Autodesk Inventor part; units mm, degrees
(part 12 of 13)
  spline S1673 degree 3 poles (16.8571, 16.1547) (16.6103, 16.1547) (16.4102, 15.9546) (16.4102, 15.7078) knots 0 0 0 0 1 1 1 1
  line L5245 (16.8571, 16.1547) -> (16.6103, 16.1547) construction
  line L5246 (16.6103, 16.1547) -> (16.4102, 15.9546) construction
  line L5247 (16.4102, 15.9546) -> (16.4102, 15.7078) construction
  spline S1674 degree 3 poles (16.4102, 15.7078) (16.4102, 15.461) (16.6103, 15.2608) (16.8571, 15.2608) knots 0 0 0 0 1 1 1 1
  line L5248 (16.4102, 15.7078) -> (16.4102, 15.461) construction
  line L5249 (16.4102, 15.461) -> (16.6103, 15.2608) construction
  line L5250 (16.6103, 15.2608) -> (16.8571, 15.2608) construction
  spline S1675 degree 3 poles (16.8571, 15.2608) (17.1039, 15.2608) (17.3041, 15.461) (17.3041, 15.7078) knots 0 0 0 0 1 1 1 1
  line L5251 (16.8571, 15.2608) -> (17.1039, 15.2608) construction
  line L5252 (17.1039, 15.2608) -> (17.3041, 15.461) construction
  line L5253 (17.3041, 15.461) -> (17.3041, 15.7078) construction
  spline S1676 degree 3 poles (17.3041, 18.2619) (17.3041, 18.5087) (17.1039, 18.7088) (16.8571, 18.7088) knots 0 0 0 0 1 1 1 1
  line L5254 (17.3041, 18.2619) -> (17.3041, 18.5087) construction
  line L5255 (17.3041, 18.5087) -> (17.1039, 18.7088) construction
  line L5256 (17.1039, 18.7088) -> (16.8571, 18.7088) construction
  spline S1677 degree 3 poles (16.8571, 18.7088) (16.6103, 18.7088) (16.4102, 18.5087) (16.4102, 18.2619) knots 0 0 0 0 1 1 1 1
  line L5257 (16.8571, 18.7088) -> (16.6103, 18.7088) construction
  line L5258 (16.6103, 18.7088) -> (16.4102, 18.5087) construction
  line L5259 (16.4102, 18.5087) -> (16.4102, 18.2619) construction
  spline S1678 degree 3 poles (16.4102, 18.2619) (16.4102, 18.0151) (16.6103, 17.8149) (16.8571, 17.8149) knots 0 0 0 0 1 1 1 1
  line L5260 (16.4102, 18.2619) -> (16.4102, 18.0151) construction
  line L5261 (16.4102, 18.0151) -> (16.6103, 17.8149) construction
  line L5262 (16.6103, 17.8149) -> (16.8571, 17.8149) construction
  spline S1679 degree 3 poles (16.8571, 17.8149) (17.1039, 17.8149) (17.3041, 18.0151) (17.3041, 18.2619) knots 0 0 0 0 1 1 1 1
  line L5263 (16.8571, 17.8149) -> (17.1039, 17.8149) construction
  line L5264 (17.1039, 17.8149) -> (17.3041, 18.0151) construction
  line L5265 (17.3041, 18.0151) -> (17.3041, 18.2619) construction
  spline S1680 degree 3 poles (17.3041, 20.816) (17.3041, 21.0628) (17.1039, 21.2629) (16.8571, 21.2629) knots 0 0 0 0 1 1 1 1
  line L5266 (17.3041, 20.816) -> (17.3041, 21.0628) construction
  line L5267 (17.3041, 21.0628) -> (17.1039, 21.2629) construction
  line L5268 (17.1039, 21.2629) -> (16.8571, 21.2629) construction
  spline S1681 degree 3 poles (16.8571, 21.2629) (16.6103, 21.2629) (16.4102, 21.0628) (16.4102, 20.816) knots 0 0 0 0 1 1 1 1
  line L5269 (16.8571, 21.2629) -> (16.6103, 21.2629) construction
  line L5270 (16.6103, 21.2629) -> (16.4102, 21.0628) construction
  line L5271 (16.4102, 21.0628) -> (16.4102, 20.816) construction
  spline S1682 degree 3 poles (16.4102, 20.816) (16.4102, 20.5692) (16.6103, 20.369) (16.8571, 20.369) knots 0 0 0 0 1 1 1 1
  line L5272 (16.4102, 20.816) -> (16.4102, 20.5692) construction
  line L5273 (16.4102, 20.5692) -> (16.6103, 20.369) construction
  line L5274 (16.6103, 20.369) -> (16.8571, 20.369) construction
  spline S1683 degree 3 poles (16.8571, 20.369) (17.1039, 20.369) (17.3041, 20.5692) (17.3041, 20.816) knots 0 0 0 0 1 1 1 1
  line L5275 (16.8571, 20.369) -> (17.1039, 20.369) construction
  line L5276 (17.1039, 20.369) -> (17.3041, 20.5692) construction
  line L5277 (17.3041, 20.5692) -> (17.3041, 20.816) construction
  spline S1684 degree 3 poles (19.8582, 13.1537) (19.8582, 13.4005) (19.658, 13.6006) (19.4112, 13.6006) knots 0 0 0 0 1 1 1 1
  line L5278 (19.8582, 13.1537) -> (19.8582, 13.4005) construction
  line L5279 (19.8582, 13.4005) -> (19.658, 13.6006) construction
  line L5280 (19.658, 13.6006) -> (19.4112, 13.6006) construction
  spline S1685 degree 3 poles (19.4112, 13.6006) (19.1644, 13.6006) (18.9643, 13.4005) (18.9643, 13.1537) knots 0 0 0 0 1 1 1 1
  line L5281 (19.4112, 13.6006) -> (19.1644, 13.6006) construction
  line L5282 (19.1644, 13.6006) -> (18.9643, 13.4005) construction
  line L5283 (18.9643, 13.4005) -> (18.9643, 13.1537) construction
  spline S1686 degree 3 poles (18.9643, 13.1537) (18.9643, 12.9069) (19.1644, 12.7067) (19.4112, 12.7067) knots 0 0 0 0 1 1 1 1
  line L5284 (18.9643, 13.1537) -> (18.9643, 12.9069) construction
  line L5285 (18.9643, 12.9069) -> (19.1644, 12.7067) construction
  line L5286 (19.1644, 12.7067) -> (19.4112, 12.7067) construction
  spline S1687 degree 3 poles (19.4112, 12.7067) (19.658, 12.7067) (19.8582, 12.9069) (19.8582, 13.1537) knots 0 0 0 0 1 1 1 1
  line L5287 (19.4112, 12.7067) -> (19.658, 12.7067) construction
  line L5288 (19.658, 12.7067) -> (19.8582, 12.9069) construction
  line L5289 (19.8582, 12.9069) -> (19.8582, 13.1537) construction
  spline S1688 degree 3 poles (19.8582, 15.7078) (19.8582, 15.9546) (19.658, 16.1547) (19.4112, 16.1547) knots 0 0 0 0 1 1 1 1
  line L5290 (19.8582, 15.7078) -> (19.8582, 15.9546) construction
  line L5291 (19.8582, 15.9546) -> (19.658, 16.1547) construction
  line L5292 (19.658, 16.1547) -> (19.4112, 16.1547) construction
  spline S1689 degree 3 poles (19.4112, 16.1547) (19.1644, 16.1547) (18.9643, 15.9546) (18.9643, 15.7078) knots 0 0 0 0 1 1 1 1
  line L5293 (19.4112, 16.1547) -> (19.1644, 16.1547) construction
  line L5294 (19.1644, 16.1547) -> (18.9643, 15.9546) construction
  line L5295 (18.9643, 15.9546) -> (18.9643, 15.7078) construction
  spline S1690 degree 3 poles (18.9643, 15.7078) (18.9643, 15.461) (19.1644, 15.2608) (19.4112, 15.2608) knots 0 0 0 0 1 1 1 1
  line L5296 (18.9643, 15.7078) -> (18.9643, 15.461) construction
  line L5297 (18.9643, 15.461) -> (19.1644, 15.2608) construction
  line L5298 (19.1644, 15.2608) -> (19.4112, 15.2608) construction
  spline S1691 degree 3 poles (19.4112, 15.2608) (19.658, 15.2608) (19.8582, 15.461) (19.8582, 15.7078) knots 0 0 0 0 1 1 1 1
  line L5299 (19.4112, 15.2608) -> (19.658, 15.2608) construction
  line L5300 (19.658, 15.2608) -> (19.8582, 15.461) construction
  line L5301 (19.8582, 15.461) -> (19.8582, 15.7078) construction
  spline S1692 degree 3 poles (19.8582, 18.2619) (19.8582, 18.5087) (19.658, 18.7088) (19.4112, 18.7088) knots 0 0 0 0 1 1 1 1
  line L5302 (19.8582, 18.2619) -> (19.8582, 18.5087) construction
  line L5303 (19.8582, 18.5087) -> (19.658, 18.7088) construction
  line L5304 (19.658, 18.7088) -> (19.4112, 18.7088) construction
  spline S1693 degree 3 poles (19.4112, 18.7088) (19.1644, 18.7088) (18.9643, 18.5087) (18.9643, 18.2619) knots 0 0 0 0 1 1 1 1
  line L5305 (19.4112, 18.7088) -> (19.1644, 18.7088) construction
  line L5306 (19.1644, 18.7088) -> (18.9643, 18.5087) construction
  line L5307 (18.9643, 18.5087) -> (18.9643, 18.2619) construction
  spline S1694 degree 3 poles (18.9643, 18.2619) (18.9643, 18.0151) (19.1644, 17.8149) (19.4112, 17.8149) knots 0 0 0 0 1 1 1 1
  line L5308 (18.9643, 18.2619) -> (18.9643, 18.0151) construction
  line L5309 (18.9643, 18.0151) -> (19.1644, 17.8149) construction
  line L5310 (19.1644, 17.8149) -> (19.4112, 17.8149) construction
  spline S1695 degree 3 poles (19.4112, 17.8149) (19.658, 17.8149) (19.8582, 18.0151) (19.8582, 18.2619) knots 0 0 0 0 1 1 1 1
  line L5311 (19.4112, 17.8149) -> (19.658, 17.8149) construction
  line L5312 (19.658, 17.8149) -> (19.8582, 18.0151) construction
  line L5313 (19.8582, 18.0151) -> (19.8582, 18.2619) construction
  spline S1696 degree 3 poles (19.8582, 20.816) (19.8582, 21.0628) (19.658, 21.2629) (19.4112, 21.2629) knots 0 0 0 0 1 1 1 1
  line L5314 (19.8582, 20.816) -> (19.8582, 21.0628) construction
  line L5315 (19.8582, 21.0628) -> (19.658, 21.2629) construction
  line L5316 (19.658, 21.2629) -> (19.4112, 21.2629) construction
  spline S1697 degree 3 poles (19.4112, 21.2629) (19.1644, 21.2629) (18.9643, 21.0628) (18.9643, 20.816) knots 0 0 0 0 1 1 1 1
  line L5317 (19.4112, 21.2629) -> (19.1644, 21.2629) construction
  line L5318 (19.1644, 21.2629) -> (18.9643, 21.0628) construction
  line L5319 (18.9643, 21.0628) -> (18.9643, 20.816) construction
  spline S1698 degree 3 poles (18.9643, 20.816) (18.9643, 20.5692) (19.1644, 20.369) (19.4112, 20.369) knots 0 0 0 0 1 1 1 1
  line L5320 (18.9643, 20.816) -> (18.9643, 20.5692) construction
  line L5321 (18.9643, 20.5692) -> (19.1644, 20.369) construction
  line L5322 (19.1644, 20.369) -> (19.4112, 20.369) construction
  spline S1699 degree 3 poles (19.4112, 20.369) (19.658, 20.369) (19.8582, 20.5692) (19.8582, 20.816) knots 0 0 0 0 1 1 1 1
  line L5323 (19.4112, 20.369) -> (19.658, 20.369) construction
  line L5324 (19.658, 20.369) -> (19.8582, 20.5692) construction
  line L5325 (19.8582, 20.5692) -> (19.8582, 20.816) construction
  spline S1700 degree 3 poles (4.0865, 32.1817) (4.0865, 32.8164) (3.5719, 33.3312) (2.9373, 33.3312) knots 0 0 0 0 1 1 1 1
  line L5326 (4.0865, 32.1817) -> (4.0865, 32.8164) construction
  line L5327 (4.0865, 32.8164) -> (3.5719, 33.3312) construction
  line L5328 (3.5719, 33.3312) -> (2.9373, 33.3312) construction
  spline S1701 degree 3 poles (2.9373, 33.3312) (2.3026, 33.3312) (1.7878, 32.8164) (1.7878, 32.1817) knots 0 0 0 0 1 1 1 1
  line L5329 (2.9373, 33.3312) -> (2.3026, 33.3312) construction
  line L5330 (2.3026, 33.3312) -> (1.7878, 32.8164) construction
  line L5331 (1.7878, 32.8164) -> (1.7878, 32.1817) construction
  spline S1702 degree 3 poles (1.7878, 32.1817) (1.7878, 31.5471) (2.3026, 31.0325) (2.9373, 31.0325) knots 0 0 0 0 1 1 1 1
  line L5332 (1.7878, 32.1817) -> (1.7878, 31.5471) construction
  line L5333 (1.7878, 31.5471) -> (2.3026, 31.0325) construction
  line L5334 (2.3026, 31.0325) -> (2.9373, 31.0325) construction
  spline S1703 degree 3 poles (2.9373, 31.0325) (3.5719, 31.0325) (4.0865, 31.5471) (4.0865, 32.1817) knots 0 0 0 0 1 1 1 1
  line L5335 (2.9373, 31.0325) -> (3.5719, 31.0325) construction
  line L5336 (3.5719, 31.0325) -> (4.0865, 31.5471) construction
  line L5337 (4.0865, 31.5471) -> (4.0865, 32.1817) construction
  spline S1704 degree 3 poles (4.0865, 1.7878) (4.0865, 2.4225) (3.5719, 2.9373) (2.9373, 2.9373) knots 0 0 0 0 1 1 1 1
  line L5338 (4.0865, 1.7878) -> (4.0865, 2.4225) construction
  line L5339 (4.0865, 2.4225) -> (3.5719, 2.9373) construction
  line L5340 (3.5719, 2.9373) -> (2.9373, 2.9373) construction
  spline S1705 degree 3 poles (2.9373, 2.9373) (2.3026, 2.9373) (1.7878, 2.4225) (1.7878, 1.7878) knots 0 0 0 0 1 1 1 1
  line L5341 (2.9373, 2.9373) -> (2.3026, 2.9373) construction
  line L5342 (2.3026, 2.9373) -> (1.7878, 2.4225) construction
  line L5343 (1.7878, 2.4225) -> (1.7878, 1.7878) construction
  spline S1706 degree 3 poles (1.7878, 1.7878) (1.7878, 1.1532) (2.3026, 0.6385) (2.9373, 0.6385) knots 0 0 0 0 1 1 1 1
  line L5344 (1.7878, 1.7878) -> (1.7878, 1.1532) construction
  line L5345 (1.7878, 1.1532) -> (2.3026, 0.6385) construction
  line L5346 (2.3026, 0.6385) -> (2.9373, 0.6385) construction
  spline S1707 degree 3 poles (2.9373, 0.6385) (3.5719, 0.6385) (4.0865, 1.1532) (4.0865, 1.7878) knots 0 0 0 0 1 1 1 1
  line L5347 (2.9373, 0.6385) -> (3.5719, 0.6385) construction
  line L5348 (3.5719, 0.6385) -> (4.0865, 1.1532) construction
  line L5349 (4.0865, 1.1532) -> (4.0865, 1.7878) construction
  spline S1708 degree 3 poles (52.3592, 1.7878) (52.3592, 2.4225) (51.8445, 2.9373) (51.2099, 2.9373) knots 0 0 0 0 1 1 1 1
  line L5350 (52.3592, 1.7878) -> (52.3592, 2.4225) construction
  line L5351 (52.3592, 2.4225) -> (51.8445, 2.9373) construction
  line L5352 (51.8445, 2.9373) -> (51.2099, 2.9373) construction
  spline S1709 degree 3 poles (51.2099, 2.9373) (50.5753, 2.9373) (50.0605, 2.4225) (50.0605, 1.7878) knots 0 0 0 0 1 1 1 1
  line L5353 (51.2099, 2.9373) -> (50.5753, 2.9373) construction
  line L5354 (50.5753, 2.9373) -> (50.0605, 2.4225) construction
  line L5355 (50.0605, 2.4225) -> (50.0605, 1.7878) construction
  spline S1710 degree 3 poles (50.0605, 1.7878) (50.0605, 1.1532) (50.5753, 0.6385) (51.2099, 0.6385) knots 0 0 0 0 1 1 1 1
  line L5356 (50.0605, 1.7878) -> (50.0605, 1.1532) construction
  line L5357 (50.0605, 1.1532) -> (50.5753, 0.6385) construction
  line L5358 (50.5753, 0.6385) -> (51.2099, 0.6385) construction
  spline S1711 degree 3 poles (51.2099, 0.6385) (51.8445, 0.6385) (52.3592, 1.1532) (52.3592, 1.7878) knots 0 0 0 0 1 1 1 1
  line L5359 (51.2099, 0.6385) -> (51.8445, 0.6385) construction
  line L5360 (51.8445, 0.6385) -> (52.3592, 1.1532) construction
  line L5361 (52.3592, 1.1532) -> (52.3592, 1.7878) construction
  spline S1712 degree 3 poles (52.3592, 32.1817) (52.3592, 32.8164) (51.8445, 33.3312) (51.2099, 33.3312) knots 0 0 0 0 1 1 1 1
  line L5362 (52.3592, 32.1817) -> (52.3592, 32.8164) construction
  line L5363 (52.3592, 32.8164) -> (51.8445, 33.3312) construction
  line L5364 (51.8445, 33.3312) -> (51.2099, 33.3312) construction
  spline S1713 degree 3 poles (51.2099, 33.3312) (50.5753, 33.3312) (50.0605, 32.8164) (50.0605, 32.1817) knots 0 0 0 0 1 1 1 1
  line L5365 (51.2099, 33.3312) -> (50.5753, 33.3312) construction
  line L5366 (50.5753, 33.3312) -> (50.0605, 32.8164) construction
  line L5367 (50.0605, 32.8164) -> (50.0605, 32.1817) construction
  spline S1714 degree 3 poles (50.0605, 32.1817) (50.0605, 31.5471) (50.5753, 31.0325) (51.2099, 31.0325) knots 0 0 0 0 1 1 1 1
  line L5368 (50.0605, 32.1817) -> (50.0605, 31.5471) construction
  line L5369 (50.0605, 31.5471) -> (50.5753, 31.0325) construction
  line L5370 (50.5753, 31.0325) -> (51.2099, 31.0325) construction
  spline S1715 degree 3 poles (51.2099, 31.0325) (51.8445, 31.0325) (52.3592, 31.5471) (52.3592, 32.1817) knots 0 0 0 0 1 1 1 1
  line L5371 (51.2099, 31.0325) -> (51.8445, 31.0325) construction
  line L5372 (51.8445, 31.0325) -> (52.3592, 31.5471) construction
  line L5373 (52.3592, 31.5471) -> (52.3592, 32.1817) construction
  line L5374 (23.6255, 14.4308) -> (23.6255, 14.1754)
  line L5375 (20.6882, 31.0325) -> (20.6882, 2.9373)
  line L5376 (18.1341, 31.0325) -> (18.1341, 2.9373)
  line L5377 (24.5194, 10.0887) -> (24.9026, 9.7057)
  line L5378 (25.6689, 10.3442) -> (26.3074, 9.7057)
  line L5379 (21.8377, 10.0887) -> (24.5194, 10.0887)
  line L5380 (21.9653, 10.3442) -> (25.6689, 10.3442)
  line L5381 (21.7099, 9.8333) -> (22.7316, 9.8333)
  line L5382 (20.6882, 10.855) -> (21.7099, 9.8333)
  line L5383 (20.4329, 10.855) -> (20.6882, 10.855)
  line L5384 (20.9436, 10.9827) -> (21.8377, 10.0887)
  line L5385 (20.9436, 12.8983) -> (20.9436, 10.9827)
  line L5386 (21.1992, 11.1103) -> (21.9653, 10.3442)
  line L5387 (20.6882, 13.1537) -> (20.9436, 12.8983)
  line L5388 (20.4329, 13.1537) -> (20.6882, 13.1537)
  line L5389 (21.1992, 15.4524) -> (21.1992, 11.1103)
  line L5390 (20.9436, 15.7078) -> (21.1992, 15.4524)
  line L5391 (20.4329, 15.7078) -> (20.9436, 15.7078)
  line L5392 (20.6882, 25.9242) -> (21.1992, 25.4133)
  line L5393 (20.4329, 25.9242) -> (20.6882, 25.9242)
  line L5394 (33.4588, 31.0325) -> (33.4588, 2.9373)
  line L5395 (36.0129, 31.0325) -> (36.0129, 2.9373)
  line L5396 (22.7316, 20.4329) -> (22.8592, 20.3051)
  line L5397 (24.6472, 20.6882) -> (24.9026, 20.4329)
  line L5398 (21.4546, 20.6882) -> (24.6472, 20.6882)
  line L5399 (21.3268, 20.4329) -> (22.7316, 20.4329)
  line L5400 (20.6882, 21.0714) -> (21.3268, 20.4329)
  line L5401 (20.4329, 21.0714) -> (20.6882, 21.0714)
  line L5402 (20.9436, 21.1992) -> (21.4546, 20.6882)
  line L5403 (25.9242, 20.9436) -> (26.3074, 20.5606)
  line L5404 (21.5822, 20.9436) -> (25.9242, 20.9436)
  line L5405 (20.9436, 23.1148) -> (20.9436, 21.1992)
  line L5406 (21.1992, 21.3268) -> (21.5822, 20.9436)
  line L5407 (21.1992, 25.4133) -> (21.1992, 21.3268)
  line L5408 (20.6882, 23.3701) -> (20.9436, 23.1148)
  spline S1716 degree 3 poles (19.4112, 32.3095) (20.1164, 32.3095) (20.6882, 31.7376) (20.6882, 31.0325) knots 0 0 0 0 1 1 1 1
  line L5409 (19.4112, 32.3095) -> (20.1164, 32.3095) construction
  line L5410 (20.1164, 32.3095) -> (20.6882, 31.7376) construction
  line L5411 (20.6882, 31.7376) -> (20.6882, 31.0325) construction
  spline S1717 degree 3 poles (18.1341, 31.0325) (18.1341, 31.7376) (18.706, 32.3095) (19.4112, 32.3095) knots 0 0 0 0 1 1 1 1
  line L5412 (18.1341, 31.0325) -> (18.1341, 31.7376) construction
  line L5413 (18.1341, 31.7376) -> (18.706, 32.3095) construction
  line L5414 (18.706, 32.3095) -> (19.4112, 32.3095) construction
  spline S1718 degree 3 poles (19.4112, 32.0541) (19.9753, 32.0541) (20.4329, 31.5966) (20.4329, 31.0325) knots 0 0 0 0 1 1 1 1
  line L5415 (19.4112, 32.0541) -> (19.9753, 32.0541) construction
  line L5416 (19.9753, 32.0541) -> (20.4329, 31.5966) construction
  line L5417 (20.4329, 31.5966) -> (20.4329, 31.0325) construction
  spline S1719 degree 3 poles (19.4112, 29.5) (19.9753, 29.5) (20.4329, 29.0425) (20.4329, 28.4784) knots 0 0 0 0 1 1 1 1
  line L5418 (19.4112, 29.5) -> (19.9753, 29.5) construction
  line L5419 (19.9753, 29.5) -> (20.4329, 29.0425) construction
  line L5420 (20.4329, 29.0425) -> (20.4329, 28.4784) construction
  spline S1720 degree 3 poles (20.4329, 28.4784) (20.4329, 27.9142) (19.9753, 27.4567) (19.4112, 27.4567) knots 0 0 0 0 1 1 1 1
  line L5421 (20.4329, 28.4784) -> (20.4329, 27.9142) construction
  line L5422 (20.4329, 27.9142) -> (19.9753, 27.4567) construction
  line L5423 (19.9753, 27.4567) -> (19.4112, 27.4567) construction
  spline S1721 degree 3 poles (20.4329, 31.0325) (20.4329, 30.4683) (19.9753, 30.0108) (19.4112, 30.0108) knots 0 0 0 0 1 1 1 1
  line L5424 (20.4329, 31.0325) -> (20.4329, 30.4683) construction
  line L5425 (20.4329, 30.4683) -> (19.9753, 30.0108) construction
  line L5426 (19.9753, 30.0108) -> (19.4112, 30.0108) construction
  spline S1722 degree 3 poles (33.4588, 31.0325) (33.4588, 31.7376) (34.0307, 32.3095) (34.7358, 32.3095) knots 0 0 0 0 1 1 1 1
  line L5427 (33.4588, 31.0325) -> (33.4588, 31.7376) construction
  line L5428 (33.4588, 31.7376) -> (34.0307, 32.3095) construction
  line L5429 (34.0307, 32.3095) -> (34.7358, 32.3095) construction
  spline S1723 degree 3 poles (34.7358, 32.3095) (35.441, 32.3095) (36.0129, 31.7376) (36.0129, 31.0325) knots 0 0 0 0 1 1 1 1
  line L5430 (34.7358, 32.3095) -> (35.441, 32.3095) construction
  line L5431 (35.441, 32.3095) -> (36.0129, 31.7376) construction
  line L5432 (36.0129, 31.7376) -> (36.0129, 31.0325) construction
  spline S1724 degree 3 poles (34.7358, 30.0108) (34.1717, 30.0108) (33.7142, 30.4683) (33.7142, 31.0325) knots 0 0 0 0 1 1 1 1
  line L5433 (34.7358, 30.0108) -> (34.1717, 30.0108) construction
  line L5434 (34.1717, 30.0108) -> (33.7142, 30.4683) construction
  line L5435 (33.7142, 30.4683) -> (33.7142, 31.0325) construction
  spline S1725 degree 3 poles (33.7142, 31.0325) (33.7142, 31.5966) (34.1717, 32.0541) (34.7358, 32.0541) knots 0 0 0 0 1 1 1 1
  line L5436 (33.7142, 31.0325) -> (33.7142, 31.5966) construction
  line L5437 (33.7142, 31.5966) -> (34.1717, 32.0541) construction
  line L5438 (34.1717, 32.0541) -> (34.7358, 32.0541) construction
  spline S1726 degree 3 poles (34.7358, 22.3485) (34.1717, 22.3485) (33.7142, 22.806) (33.7142, 23.3701) knots 0 0 0 0 1 1 1 1
  line L5439 (34.7358, 22.3485) -> (34.1717, 22.3485) construction
  line L5440 (34.1717, 22.3485) -> (33.7142, 22.806) construction
  line L5441 (33.7142, 22.806) -> (33.7142, 23.3701) construction
  spline S1727 degree 3 poles (33.7142, 23.3701) (33.7142, 23.9342) (34.1717, 24.3918) (34.7358, 24.3918) knots 0 0 0 0 1 1 1 1
  line L5442 (33.7142, 23.3701) -> (33.7142, 23.9342) construction
  line L5443 (33.7142, 23.9342) -> (34.1717, 24.3918) construction
  line L5444 (34.1717, 24.3918) -> (34.7358, 24.3918) construction
  spline S1728 degree 3 poles (34.7358, 19.7943) (34.1717, 19.7943) (33.7142, 20.2519) (33.7142, 20.816) knots 0 0 0 0 1 1 1 1
  line L5445 (34.7358, 19.7943) -> (34.1717, 19.7943) construction
  line L5446 (34.1717, 19.7943) -> (33.7142, 20.2519) construction
  line L5447 (33.7142, 20.2519) -> (33.7142, 20.816) construction
  spline S1729 degree 3 poles (33.7142, 20.816) (33.7142, 21.3801) (34.1717, 21.8377) (34.7358, 21.8377) knots 0 0 0 0 1 1 1 1
  line L5448 (33.7142, 20.816) -> (33.7142, 21.3801) construction
  line L5449 (33.7142, 21.3801) -> (34.1717, 21.8377) construction
  line L5450 (34.1717, 21.8377) -> (34.7358, 21.8377) construction
  spline S1730 degree 3 poles (34.7358, 14.6861) (34.1717, 14.6861) (33.7142, 15.1437) (33.7142, 15.7078) knots 0 0 0 0 1 1 1 1
  line L5451 (34.7358, 14.6861) -> (34.1717, 14.6861) construction
  line L5452 (34.1717, 14.6861) -> (33.7142, 15.1437) construction
  line L5453 (33.7142, 15.1437) -> (33.7142, 15.7078) construction
  spline S1731 degree 3 poles (33.7142, 15.7078) (33.7142, 16.2719) (34.1717, 16.7295) (34.7358, 16.7295) knots 0 0 0 0 1 1 1 1
  line L5454 (33.7142, 15.7078) -> (33.7142, 16.2719) construction
  line L5455 (33.7142, 16.2719) -> (34.1717, 16.7295) construction
  line L5456 (34.1717, 16.7295) -> (34.7358, 16.7295) construction
  spline S1732 degree 3 poles (20.6882, 2.9373) (20.6882, 2.2321) (20.1164, 1.6602) (19.4112, 1.6602) knots 0 0 0 0 1 1 1 1
  line L5457 (20.6882, 2.9373) -> (20.6882, 2.2321) construction
  line L5458 (20.6882, 2.2321) -> (20.1164, 1.6602) construction
  line L5459 (20.1164, 1.6602) -> (19.4112, 1.6602) construction
  spline S1733 degree 3 poles (19.4112, 1.6602) (18.706, 1.6602) (18.1341, 2.2321) (18.1341, 2.9373) knots 0 0 0 0 1 1 1 1
  line L5460 (19.4112, 1.6602) -> (18.706, 1.6602) construction
  line L5461 (18.706, 1.6602) -> (18.1341, 2.2321) construction
  line L5462 (18.1341, 2.2321) -> (18.1341, 2.9373) construction
  spline S1734 degree 3 poles (34.7358, 1.6602) (34.0307, 1.6602) (33.4588, 2.2321) (33.4588, 2.9373) knots 0 0 0 0 1 1 1 1
  line L5463 (34.7358, 1.6602) -> (34.0307, 1.6602) construction
  line L5464 (34.0307, 1.6602) -> (33.4588, 2.2321) construction
  line L5465 (33.4588, 2.2321) -> (33.4588, 2.9373) construction
  spline S1735 degree 3 poles (36.0129, 2.9373) (36.0129, 2.2321) (35.441, 1.6602) (34.7358, 1.6602) knots 0 0 0 0 1 1 1 1
  line L5466 (36.0129, 2.9373) -> (36.0129, 2.2321) construction
  line L5467 (36.0129, 2.2321) -> (35.441, 1.6602) construction
  line L5468 (35.441, 1.6602) -> (34.7358, 1.6602) construction
  line L5469 (20.4329, 23.3701) -> (20.6882, 23.3701)
  line L5470 (27.1247, 13.7922) -> (26.5116, 13.7922)
  line L5471 (27.3289, 13.9352) -> (27.1247, 13.7922)
  line L5472 (27.3289, 14.16) -> (27.3289, 13.9352)
  line L5473 (27.1247, 14.303) -> (27.3289, 14.16)
  line L5474 (27.1247, 14.303) -> (26.5116, 14.303)
  line L5475 (26.9203, 14.303) -> (26.9203, 13.7922)
  line L5476 (27.3289, 14.9569) -> (26.8181, 14.5482)
  line L5477 (26.8181, 15.059) -> (26.8181, 14.5482)
  line L5478 (27.3289, 14.9569) -> (26.5116, 14.9569)
  line L5479 (27.1247, 21.7099) -> (26.5116, 21.7099)
  line L5480 (27.3289, 21.8529) -> (27.1247, 21.7099)
  line L5481 (27.3289, 22.0777) -> (27.3289, 21.8529)
  line L5482 (27.1247, 22.2207) -> (27.3289, 22.0777)
  line L5483 (27.1247, 22.2207) -> (26.5116, 22.2207)
  line L5484 (26.9203, 22.2207) -> (26.9203, 21.7099)
  line L5485 (27.3289, 22.9767) -> (26.5116, 22.5681)
  line L5486 (27.3289, 22.9767) -> (27.3289, 22.4659)
  line L5487 (27.1247, 24.264) -> (26.5116, 24.264)
  line L5488 (27.3289, 24.407) -> (27.1247, 24.264)
  line L5489 (27.3289, 24.6318) -> (27.3289, 24.407)
  line L5490 (27.1247, 24.7748) -> (27.3289, 24.6318)
  line L5491 (27.1247, 24.7748) -> (26.5116, 24.7748)
  line L5492 (26.9203, 24.7748) -> (26.9203, 24.264)
  line L5493 (27.2268, 25.4287) -> (27.3289, 25.3266)
  line L5494 (27.3289, 25.3266) -> (27.3289, 25.1222)
  line L5495 (27.3289, 25.1222) -> (27.2268, 25.0201)
  line L5496 (27.2268, 25.0201) -> (26.6137, 25.0201)
  line L5497 (26.5116, 25.1222) -> (26.6137, 25.0201)
  line L5498 (26.859, 25.4287) -> (26.9611, 25.3266)
  line L5499 (26.9611, 25.3266) -> (26.9611, 25.0201)
  line L5500 (26.5116, 25.3266) -> (26.5116, 25.1222)
  line L5501 (26.6137, 25.4287) -> (26.5116, 25.3266)
  line L5502 (26.859, 25.4287) -> (26.6137, 25.4287)
  line L5503 (21.8887, 17.751) -> (21.2758, 17.751)
  line L5504 (22.0931, 17.8942) -> (21.8887, 17.751)
  line L5505 (22.0931, 18.1189) -> (22.0931, 17.8942)
  line L5506 (21.8887, 18.2619) -> (22.0931, 18.1189)
  line L5507 (21.8887, 18.2619) -> (21.2758, 18.2619)
  line L5508 (21.6844, 18.2619) -> (21.6844, 17.751)
  line L5509 (22.0931, 18.6705) -> (21.9295, 18.507)
  line L5510 (22.0931, 18.6705) -> (21.2758, 18.6705)
  line L5511 (21.2758, 18.8136) -> (21.2758, 18.507)
  line L5512 (23.6766, 19.1558) -> (23.0636, 19.1558)
  line L5513 (23.8809, 19.2988) -> (23.6766, 19.1558)
  line L5514 (23.8809, 19.5236) -> (23.8809, 19.2988)
  line L5515 (23.6766, 19.6666) -> (23.8809, 19.5236)
  line L5516 (23.6766, 19.6666) -> (23.0636, 19.6666)
  line L5517 (23.4723, 19.6666) -> (23.4723, 19.1558)
  line L5518 (23.0636, 20.014) -> (23.1657, 19.9118)
  line L5519 (23.7788, 19.9118) -> (23.1657, 19.9118)
  line L5520 (23.8809, 20.014) -> (23.7788, 19.9118)
  line L5521 (23.8809, 20.2184) -> (23.8809, 20.014)
  line L5522 (23.7788, 20.3205) -> (23.8809, 20.2184)
  line L5523 (23.7788, 20.3205) -> (23.1657, 20.3205)
  line L5524 (23.1657, 20.3205) -> (23.0636, 20.2184)
  line L5525 (23.0636, 20.2184) -> (23.0636, 20.014)
  line L5526 (23.6766, 20.3205) -> (23.268, 19.9118)
  line L5527 (25.2857, 19.3193) -> (25.1222, 19.1558)
  line L5528 (25.2857, 19.3193) -> (24.4684, 19.3193)
  line L5529 (24.4684, 19.4623) -> (24.4684, 19.1558)
  line L5530 (25.2857, 19.8097) -> (25.1836, 19.7075)
  line L5531 (25.2857, 20.014) -> (25.2857, 19.8097)
  line L5532 (25.1836, 20.1161) -> (25.2857, 20.014)
  line L5533 (24.5706, 20.1161) -> (24.4684, 20.014)
  line L5534 (24.4684, 20.014) -> (24.4684, 19.8097)
  line L5535 (24.4684, 19.8097) -> (24.5706, 19.7075)
  line L5536 (24.918, 20.014) -> (24.918, 19.8097)
  line L5537 (25.1836, 20.1161) -> (25.0201, 20.1161)
  line L5538 (24.8157, 20.1161) -> (24.5706, 20.1161)
  line L5539 (24.918, 20.014) -> (24.8157, 20.1161)
  line L5540 (24.918, 20.014) -> (25.0201, 20.1161)
  line L5541 (26.6904, 19.3193) -> (26.527, 19.1558)
  line L5542 (26.6904, 19.3193) -> (25.8731, 19.3193)
  line L5543 (25.8731, 19.4623) -> (25.8731, 19.1558)
  line L5544 (26.6904, 19.8097) -> (26.5883, 19.7075)
  line L5545 (26.6904, 20.1161) -> (26.6904, 19.8097)
  line L5546 (26.5883, 20.2184) -> (26.6904, 20.1161)
  line L5547 (26.5883, 20.2184) -> (26.384, 20.2184)
  line L5548 (26.384, 20.2184) -> (25.8731, 19.7075)
  line L5549 (25.8731, 20.2184) -> (25.8731, 19.7075)
  line L5550 (22.0931, 30.8128) -> (21.9295, 30.6493)
  line L5551 (22.0931, 30.8128) -> (21.2758, 30.8128)
  line L5552 (21.2758, 30.9558) -> (21.2758, 30.6493)
  line L5553 (21.2758, 31.3032) -> (21.3779, 31.201)
  line L5554 (21.991, 31.201) -> (21.3779, 31.201)
  line L5555 (22.0931, 31.3032) -> (21.991, 31.201)
  line L5556 (22.0931, 31.5075) -> (22.0931, 31.3032)
  line L5557 (21.991, 31.6096) -> (22.0931, 31.5075)
  line L5558 (21.991, 31.6096) -> (21.3779, 31.6096)
  line L5559 (21.3779, 31.6096) -> (21.2758, 31.5075)
  line L5560 (21.2758, 31.5075) -> (21.2758, 31.3032)
  line L5561 (21.8887, 31.6096) -> (21.4801, 31.201)
  line L5562 (22.0931, 28.2587) -> (21.9295, 28.0952)
  line L5563 (22.0931, 28.2587) -> (21.2758, 28.2587)
  line L5564 (21.2758, 28.4017) -> (21.2758, 28.0952)
  line L5565 (22.0931, 28.8104) -> (21.9295, 28.6469)
  line L5566 (22.0931, 28.8104) -> (21.2758, 28.8104)
  line L5567 (21.2758, 28.9533) -> (21.2758, 28.6469)
  line L5568 (32.0541, 15.8611) -> (32.1562, 15.9632)
  line L5569 (32.0541, 15.8611) -> (32.0541, 15.6567)
  line L5570 (32.1562, 15.5545) -> (32.0541, 15.6567)
  line L5571 (32.7693, 15.5545) -> (32.8714, 15.6567)
  line L5572 (32.8714, 15.8611) -> (32.8714, 15.6567)
  line L5573 (32.8714, 15.8611) -> (32.7693, 15.9632)
  line L5574 (32.4219, 15.8611) -> (32.4219, 15.6567)
  line L5575 (32.3198, 15.5545) -> (32.1562, 15.5545)
  line L5576 (32.7693, 15.5545) -> (32.524, 15.5545)
  line L5577 (32.4219, 15.6567) -> (32.524, 15.5545)
  line L5578 (32.4219, 15.6567) -> (32.3198, 15.5545)
  line L5579 (32.0541, 18.1086) -> (32.5649, 18.5173)
  line L5580 (32.5649, 18.5173) -> (32.5649, 18.0065)
  line L5581 (32.8714, 18.1086) -> (32.0541, 18.1086)
  line L5582 (32.1562, 23.2169) -> (32.0541, 23.319)
  line L5583 (32.0541, 23.5234) -> (32.0541, 23.319)
  line L5584 (32.0541, 23.5234) -> (32.1562, 23.6255)
  line L5585 (32.7693, 23.6255) -> (32.1562, 23.6255)
  line L5586 (32.8714, 23.5234) -> (32.7693, 23.6255)
  line L5587 (32.524, 23.2169) -> (32.4219, 23.319)
  line L5588 (32.4219, 23.6255) -> (32.4219, 23.319)
  line L5589 (32.8714, 23.5234) -> (32.8714, 23.319)
  line L5590 (32.7693, 23.2169) -> (32.8714, 23.319)
  line L5591 (32.7693, 23.2169) -> (32.524, 23.2169)
  line L5592 (32.0541, 13.3069) -> (32.1562, 13.4091)
  line L5593 (32.0541, 13.3069) -> (32.0541, 13.0004)
  line L5594 (32.1562, 12.8983) -> (32.0541, 13.0004)
  line L5595 (32.3605, 12.8983) -> (32.1562, 12.8983)
  line L5596 (32.3605, 12.8983) -> (32.8714, 13.4091)
  line L5597 (32.8714, 13.4091) -> (32.8714, 12.8983)
  line L5598 (32.0541, 21.0714) -> (32.0541, 20.6627)
  line L5599 (32.4628, 21.0714) -> (32.0541, 21.0714)
  line L5600 (32.3605, 20.9693) -> (32.4628, 21.0714)
  line L5601 (32.3605, 20.9693) -> (32.3605, 20.7649)
  line L5602 (32.4628, 20.6627) -> (32.3605, 20.7649)
  line L5603 (32.7693, 20.6627) -> (32.4628, 20.6627)
  line L5604 (32.7693, 20.6627) -> (32.8714, 20.7649)
  line L5605 (32.8714, 20.9693) -> (32.8714, 20.7649)
  line L5606 (32.8714, 20.9693) -> (32.7693, 21.0714)
  line L5607 (32.0541, 25.6689) -> (32.8714, 26.0775)
  line L5608 (32.0541, 26.1796) -> (32.0541, 25.6689)
  line L5609 (32.8714, 28.6316) -> (32.7693, 28.7337)
  line L5610 (32.7693, 28.7337) -> (32.6058, 28.7337)
  line L5611 (32.4628, 28.5907) -> (32.6058, 28.7337)
  line L5612 (32.4628, 28.5907) -> (32.4628, 28.4681)
  line L5613 (32.6058, 28.3251) -> (32.4628, 28.4681)
  line L5614 (32.7693, 28.3251) -> (32.6058, 28.3251)
  line L5615 (32.7693, 28.3251) -> (32.8714, 28.4272)
  line L5616 (32.8714, 28.6316) -> (32.8714, 28.4272)
  line L5617 (32.4628, 28.5907) -> (32.3198, 28.7337)
  line L5618 (32.3198, 28.7337) -> (32.1562, 28.7337)
  line L5619 (32.0541, 28.6316) -> (32.1562, 28.7337)
  line L5620 (32.0541, 28.6316) -> (32.0541, 28.4272)
  line L5621 (32.1562, 28.3251) -> (32.0541, 28.4272)
  line L5622 (32.3198, 28.3251) -> (32.1562, 28.3251)
  line L5623 (32.3198, 28.3251) -> (32.4628, 28.4681)
  line L5624 (32.4628, 30.8792) -> (32.8714, 31.1857)
  line L5625 (32.4628, 30.8792) -> (32.1562, 30.8792)
  line L5626 (32.1562, 30.8792) -> (32.0541, 30.9813)
  line L5627 (32.0541, 31.1857) -> (32.0541, 30.9813)
  line L5628 (32.0541, 31.1857) -> (32.1562, 31.2878)
  line L5629 (32.3605, 31.2878) -> (32.1562, 31.2878)
  line L5630 (32.4628, 31.1857) -> (32.3605, 31.2878)
  line L5631 (32.4628, 31.1857) -> (32.4628, 30.8792)
  line L5632 (26.4861, 8.1731) -> (25.8731, 8.1731)
  line L5633 (26.6904, 8.3163) -> (26.4861, 8.1731)
  line L5634 (26.6904, 8.541) -> (26.6904, 8.3163)
  line L5635 (26.4861, 8.684) -> (26.6904, 8.541)
  line L5636 (26.4861, 8.684) -> (25.8731, 8.684)
  line L5637 (26.2817, 8.684) -> (26.2817, 8.1731)
  line L5638 (26.6904, 9.0314) -> (26.5883, 8.9291)
  line L5639 (26.6904, 9.3378) -> (26.6904, 9.0314)
  line L5640 (26.5883, 9.44) -> (26.6904, 9.3378)
  line L5641 (26.5883, 9.44) -> (26.384, 9.44)
  line L5642 (26.384, 9.44) -> (25.8731, 8.9291)
  line L5643 (25.8731, 9.44) -> (25.8731, 8.9291)
  line L5644 (25.0813, 8.1731) -> (24.4684, 8.1731)
  line L5645 (25.2857, 8.3163) -> (25.0813, 8.1731)
  line L5646 (25.2857, 8.541) -> (25.2857, 8.3163)
  line L5647 (25.0813, 8.684) -> (25.2857, 8.541)
  line L5648 (25.0813, 8.684) -> (24.4684, 8.684)
  line L5649 (24.8771, 8.684) -> (24.8771, 8.1731)
  line L5650 (25.2857, 9.0314) -> (25.1836, 8.9291)
  line L5651 (25.2857, 9.2357) -> (25.2857, 9.0314)
  line L5652 (25.1836, 9.3378) -> (25.2857, 9.2357)
  line L5653 (24.5706, 9.3378) -> (24.4684, 9.2357)
  line L5654 (24.4684, 9.2357) -> (24.4684, 9.0314)
  line L5655 (24.4684, 9.0314) -> (24.5706, 8.9291)
  line L5656 (24.918, 9.2357) -> (24.918, 9.0314)
  line L5657 (25.1836, 9.3378) -> (25.0201, 9.3378)
  line L5658 (24.8157, 9.3378) -> (24.5706, 9.3378)
  line L5659 (24.918, 9.2357) -> (24.8157, 9.3378)
  line L5660 (24.918, 9.2357) -> (25.0201, 9.3378)
  line L5661 (23.0636, 8.3775) -> (23.8809, 8.1731)
  line L5662 (23.8809, 8.5819) -> (23.0636, 8.3775)
  line L5663 (23.0636, 9.2357) -> (23.0636, 8.97)
  line L5664 (23.0636, 8.97) -> (23.2066, 8.827)
  line L5665 (23.7379, 8.827) -> (23.2066, 8.827)
  line L5666 (23.8809, 8.97) -> (23.7379, 8.827)
  line L5667 (23.8809, 9.2357) -> (23.8809, 8.97)
  line L5668 (23.0636, 9.8895) -> (23.0636, 9.6239)
  line L5669 (23.0636, 9.6239) -> (23.2066, 9.4809)
  line L5670 (23.7379, 9.4809) -> (23.2066, 9.4809)
  line L5671 (23.8809, 9.6239) -> (23.7379, 9.4809)
  line L5672 (23.8809, 9.8895) -> (23.8809, 9.6239)
  line L5673 (27.1247, 11.2381) -> (26.5116, 11.2381)
  line L5674 (27.3289, 11.3811) -> (27.1247, 11.2381)
  line L5675 (27.3289, 11.6059) -> (27.3289, 11.3811)
  line L5676 (27.1247, 11.7489) -> (27.3289, 11.6059)
  line L5677 (27.1247, 11.7489) -> (26.5116, 11.7489)
  line L5678 (26.9203, 11.7489) -> (26.9203, 11.2381)
  line L5679 (27.3289, 12.4028) -> (27.3289, 11.9941)
  line L5680 (27.3289, 11.9941) -> (26.9203, 11.9941)
  line L5681 (27.0225, 12.0963) -> (26.9203, 11.9941)
  line L5682 (27.0225, 12.3007) -> (27.0225, 12.0963)
  line L5683 (26.9203, 12.4028) -> (27.0225, 12.3007)
  line L5684 (26.9203, 12.4028) -> (26.6137, 12.4028)
  line L5685 (26.6137, 12.4028) -> (26.5116, 12.3007)
  line L5686 (26.5116, 12.3007) -> (26.5116, 12.0963)
  line L5687 (26.5116, 12.0963) -> (26.6137, 11.9941)
  line L5688 (22.0931, 2.3242) -> (22.0931, 1.9156)
  line L5689 (21.991, 2.4263) -> (22.0931, 2.3242)
  line L5690 (21.991, 2.4263) -> (21.7866, 2.4263)
  line L5691 (21.7866, 2.4263) -> (21.6844, 2.3242)
  line L5692 (21.6844, 2.3242) -> (21.6844, 2.0177)
  line L5693 (22.0931, 2.0177) -> (21.2758, 2.0177)
  line L5694 (21.2758, 2.4263) -> (21.6844, 2.1812)
  line L5695 (21.8887, 2.6716) -> (21.2758, 2.6716)
  line L5696 (22.0931, 2.8146) -> (21.8887, 2.6716)
  line L5697 (22.0931, 3.0394) -> (22.0931, 2.8146)
  line L5698 (21.8887, 3.1824) -> (22.0931, 3.0394)
  line L5699 (21.8887, 3.1824) -> (21.2758, 3.1824)
  line L5700 (21.6844, 3.1824) -> (21.6844, 2.6716)
  line L5701 (22.0931, 3.4276) -> (21.6844, 3.4276)
  line L5702 (21.2758, 3.5298) -> (21.6844, 3.4276)
  line L5703 (21.6844, 3.7342) -> (21.2758, 3.5298)
  line L5704 (21.2758, 3.9384) -> (21.6844, 3.7342)
  line L5705 (21.6844, 4.0405) -> (21.2758, 3.9384)
  line L5706 (22.0931, 4.0405) -> (21.6844, 4.0405)
  line L5707 (21.991, 4.9804) -> (22.0931, 4.8783)
  line L5708 (22.0931, 4.8783) -> (22.0931, 4.5718)
  line L5709 (22.0931, 4.5718) -> (21.991, 4.4697)
  line L5710 (21.991, 4.4697) -> (21.3779, 4.4697)
  line L5711 (21.2758, 4.5718) -> (21.3779, 4.4697)
  line L5712 (21.2758, 4.8783) -> (21.2758, 4.5718)
  line L5713 (21.3779, 4.9804) -> (21.2758, 4.8783)
  line L5714 (21.5822, 4.9804) -> (21.3779, 4.9804)
  line L5715 (21.5822, 4.9804) -> (21.6844, 4.8783)
  line L5716 (21.6844, 4.8783) -> (21.6844, 4.6741)
  line L5717 (22.0931, 5.2257) -> (21.2758, 5.2257)
  line L5718 (21.2758, 5.7365) -> (22.0931, 5.2257)
  line L5719 (22.0931, 5.7365) -> (21.2758, 5.7365)
  line L5720 (22.0931, 6.0839) -> (21.2758, 6.0839)
  line L5721 (21.9501, 6.4925) -> (22.0931, 6.3495)
  line L5722 (21.9501, 6.4925) -> (21.4188, 6.4925)
  line L5723 (21.4188, 6.4925) -> (21.2758, 6.3495)
  line L5724 (21.2758, 6.3495) -> (21.2758, 5.9818)
  line L5725 (22.0931, 6.3495) -> (22.0931, 5.9818)
  line L5726 (22.0931, 7.4325) -> (22.0931, 7.0238)
  line L5727 (21.991, 7.5346) -> (22.0931, 7.4325)
  line L5728 (21.991, 7.5346) -> (21.7866, 7.5346)
  line L5729 (21.7866, 7.5346) -> (21.6844, 7.4325)
  line L5730 (21.6844, 7.4325) -> (21.6844, 7.1259)
  line L5731 (22.0931, 7.1259) -> (21.2758, 7.1259)
  line L5732 (21.2758, 7.5346) -> (21.6844, 7.2894)
  line L5733 (21.991, 8.2906) -> (22.0931, 8.1885)
  line L5734 (22.0931, 8.1885) -> (22.0931, 7.8819)
  line L5735 (22.0931, 7.8819) -> (21.991, 7.7798)
  line L5736 (21.991, 7.7798) -> (21.7866, 7.7798)
  line L5737 (21.6844, 7.8819) -> (21.7866, 7.7798)
  line L5738 (21.6844, 8.1885) -> (21.6844, 7.8819)
  line L5739 (21.5822, 8.2906) -> (21.6844, 8.1885)
  line L5740 (21.5822, 8.2906) -> (21.3779, 8.2906)
  line L5741 (21.3779, 8.2906) -> (21.2758, 8.1885)
  line L5742 (21.2758, 8.1885) -> (21.2758, 7.8819)
  line L5743 (21.2758, 7.8819) -> (21.3779, 7.7798)
  line L5744 (22.0931, 8.9445) -> (22.0931, 8.5359)
  line L5745 (22.0931, 8.7401) -> (21.2758, 8.7401)
  line L5746 (25.3878, 1.6091) -> (24.9792, 1.6091)
  line L5747 (25.49, 1.7112) -> (25.3878, 1.6091)
  line L5748 (25.49, 1.9156) -> (25.49, 1.7112)
  line L5749 (25.49, 1.9156) -> (25.3878, 2.0177)
  line L5750 (25.3878, 2.0177) -> (25.0813, 2.0177)
  line L5751 (25.0813, 2.4263) -> (25.0813, 1.6091)
  line L5752 (25.49, 2.4263) -> (25.2448, 2.0177)
  line L5753 (26.246, 1.6091) -> (25.7352, 2.4263)
  line L5754 (26.246, 2.4263) -> (25.7352, 1.6091)
  line L5755 (26.6955, 1.6091) -> (26.4913, 1.6091)
  line L5756 (26.5934, 2.4263) -> (26.5934, 1.6091)
  line L5757 (26.6955, 2.4263) -> (26.4913, 2.4263)
  line L5758 (19.4368, -0.1278) -> (19.539, -0.2299)
  line L5759 (19.539, -0.2299) -> (19.539, -0.5364)
  line L5760 (19.539, -0.5364) -> (19.4368, -0.6385)
  line L5761 (19.4368, -0.6385) -> (18.8238, -0.6385)
  line L5762 (18.7217, -0.5364) -> (18.8238, -0.6385)
  line L5763 (18.7217, -0.2299) -> (18.7217, -0.5364)
  line L5764 (18.8238, -0.1278) -> (18.7217, -0.2299)
  line L5765 (19.028, -0.1278) -> (18.8238, -0.1278)
  line L5766 (19.028, -0.1278) -> (19.1303, -0.2299)
  line L5767 (19.1303, -0.2299) -> (19.1303, -0.4342)
  line L5768 (19.539, 0.5261) -> (19.539, 0.1175)
  line L5769 (19.4368, 0.6283) -> (19.539, 0.5261)
  line L5770 (19.4368, 0.6283) -> (19.2324, 0.6283)
  line L5771 (19.2324, 0.6283) -> (19.1303, 0.5261)
  line L5772 (19.1303, 0.5261) -> (19.1303, 0.2196)
  line L5773 (19.539, 0.2196) -> (18.7217, 0.2196)
  line L5774 (18.7217, 0.6283) -> (19.1303, 0.3832)
  line L5775 (19.539, 0.8735) -> (18.7217, 0.8735)
  line L5776 (18.7217, 1.3843) -> (19.539, 0.8735)
  line L5777 (19.539, 1.3843) -> (18.7217, 1.3843)
  line L5778 (23.0125, 1.6091) -> (22.6038, 1.6091)
  line L5779 (22.8082, 2.4263) -> (22.8082, 1.6091)
  line L5780 (23.7685, 1.6091) -> (23.2578, 2.4263)
  line L5781 (23.7685, 2.4263) -> (23.2578, 1.6091)
  line L5782 (24.0138, 2.3242) -> (24.0138, 1.7112)
  line L5783 (24.1159, 1.6091) -> (24.0138, 1.7112)
  line L5784 (24.3203, 1.6091) -> (24.1159, 1.6091)
  line L5785 (24.4224, 1.7112) -> (24.3203, 1.6091)
  line L5786 (24.4224, 2.3242) -> (24.4224, 1.7112)
  line L5787 (24.4224, 2.3242) -> (24.3203, 2.4263)
  line L5788 (24.3203, 2.4263) -> (24.1159, 2.4263)
  line L5789 (24.1159, 2.4263) -> (24.0138, 2.3242)
  line L5790 (32.0541, 9.0672) -> (32.0541, 8.6584)
  line L5791 (32.1562, 8.5562) -> (32.0541, 8.6584)
  line L5792 (32.3605, 8.5562) -> (32.1562, 8.5562)
  line L5793 (32.3605, 8.5562) -> (32.4628, 8.6584)
  line L5794 (32.4628, 8.9649) -> (32.4628, 8.6584)
  line L5795 (32.8714, 8.9649) -> (32.0541, 8.9649)
  line L5796 (32.8714, 8.5562) -> (32.4628, 8.8015)
  line L5797 (32.1562, 7.8002) -> (32.0541, 7.9025)
  line L5798 (32.0541, 8.2088) -> (32.0541, 7.9025)
  line L5799 (32.0541, 8.2088) -> (32.1562, 8.3111)
  line L5800 (32.3605, 8.3111) -> (32.1562, 8.3111)
  line L5801 (32.4628, 8.2088) -> (32.3605, 8.3111)
  line L5802 (32.4628, 8.2088) -> (32.4628, 7.9025)
  line L5803 (32.5649, 7.8002) -> (32.4628, 7.9025)
  line L5804 (32.7693, 7.8002) -> (32.5649, 7.8002)
  line L5805 (32.7693, 7.8002) -> (32.8714, 7.9025)
  line L5806 (32.8714, 8.2088) -> (32.8714, 7.9025)
  line L5807 (32.8714, 8.2088) -> (32.7693, 8.3111)
  line L5808 (32.0541, 7.5551) -> (32.0541, 7.1464)
  line L5809 (32.8714, 7.3507) -> (32.0541, 7.3507)
  line L5810 (32.1562, 11.1103) -> (32.0541, 11.2125)
  line L5811 (32.0541, 11.519) -> (32.0541, 11.2125)
  line L5812 (32.0541, 11.519) -> (32.1562, 11.6213)
  line L5813 (32.7693, 11.6213) -> (32.1562, 11.6213)
  line L5814 (32.8714, 11.519) -> (32.7693, 11.6213)
  line L5815 (32.8714, 11.519) -> (32.8714, 11.2125)
  line L5816 (32.7693, 11.1103) -> (32.8714, 11.2125)
  line L5817 (32.7693, 11.1103) -> (32.5649, 11.1103)
  line L5818 (32.5649, 11.1103) -> (32.4628, 11.2125)
  line L5819 (32.4628, 11.4169) -> (32.4628, 11.2125)
  line L5820 (32.8714, 10.8652) -> (32.0541, 10.8652)
  line L5821 (32.8714, 10.3543) -> (32.0541, 10.8652)
  line L5822 (32.8714, 10.3543) -> (32.0541, 10.3543)
  line L5823 (32.8714, 10.0071) -> (32.0541, 10.0071)
  line L5824 (32.1971, 9.5983) -> (32.0541, 9.7414)
  line L5825 (32.7284, 9.5983) -> (32.1971, 9.5983)
  line L5826 (32.7284, 9.5983) -> (32.8714, 9.7414)
  line L5827 (32.8714, 10.1092) -> (32.8714, 9.7414)
  line L5828 (32.0541, 10.1092) -> (32.0541, 9.7414)
  line L5829 (32.0541, 3.8312) -> (32.0541, 3.4225)
  line L5830 (32.8714, 3.6268) -> (32.0541, 3.6268)
  line L5831 (32.0541, 2.6665) -> (32.8714, 3.1772)
  line L5832 (32.8714, 2.6665) -> (32.0541, 3.1772)
  line L5833 (32.7693, 2.4214) -> (32.1562, 2.4214)
  line L5834 (32.0541, 2.3191) -> (32.1562, 2.4214)
  line L5835 (32.0541, 2.3191) -> (32.0541, 2.1148)
  line L5836 (32.1562, 2.0126) -> (32.0541, 2.1148)
  line L5837 (32.7693, 2.0126) -> (32.1562, 2.0126)
  line L5838 (32.7693, 2.0126) -> (32.8714, 2.1148)
  line L5839 (32.8714, 2.3191) -> (32.8714, 2.1148)
  line L5840 (32.8714, 2.3191) -> (32.7693, 2.4214)
  line L5841 (32.0541, 6.3853) -> (32.0541, 5.9766)
  line L5842 (32.1562, 5.8745) -> (32.0541, 5.9766)
  line L5843 (32.3605, 5.8745) -> (32.1562, 5.8745)
  line L5844 (32.3605, 5.8745) -> (32.4628, 5.9766)
  line L5845 (32.4628, 6.2831) -> (32.4628, 5.9766)
  line L5846 (32.8714, 6.2831) -> (32.0541, 6.2831)
  line L5847 (32.8714, 5.8745) -> (32.4628, 6.1196)
  line L5848 (32.0541, 5.1185) -> (32.8714, 5.6292)
  line L5849 (32.8714, 5.1185) -> (32.0541, 5.6292)
  line L5850 (32.0541, 4.8732) -> (32.0541, 4.6689)
  line L5851 (32.8714, 4.7711) -> (32.0541, 4.7711)
  line L5852 (32.8714, 4.8732) -> (32.8714, 4.6689)
  line L5853 (30.0363, 1.7112) -> (29.9342, 1.6091)
  line L5854 (29.9342, 1.6091) -> (29.6276, 1.6091)
  line L5855 (29.6276, 1.6091) -> (29.5255, 1.7112)
  line L5856 (29.5255, 2.3242) -> (29.5255, 1.7112)
  line L5857 (29.6276, 2.4263) -> (29.5255, 2.3242)
  line L5858 (29.9342, 2.4263) -> (29.6276, 2.4263)
  line L5859 (30.0363, 2.3242) -> (29.9342, 2.4263)
  line L5860 (30.0363, 2.3242) -> (30.0363, 2.12)
  line L5861 (30.0363, 2.12) -> (29.9342, 2.0177)
  line L5862 (29.9342, 2.0177) -> (29.7298, 2.0177)
  line L5863 (30.2816, 2.4263) -> (30.2816, 1.6091)
  line L5864 (30.7923, 2.4263) -> (30.2816, 1.6091)
  line L5865 (30.7923, 2.4263) -> (30.7923, 1.6091)
  line L5866 (31.1397, 2.4263) -> (31.1397, 1.6091)
  line L5867 (31.5484, 1.7521) -> (31.4054, 1.6091)
  line L5868 (31.5484, 2.2833) -> (31.5484, 1.7521)
  line L5869 (31.5484, 2.2833) -> (31.4054, 2.4263)
  line L5870 (31.4054, 2.4263) -> (31.0376, 2.4263)
  line L5871 (31.4054, 1.6091) -> (31.0376, 1.6091)
  line L5872 (27.6099, 2.4263) -> (27.4056, 1.6091)
  line L5873 (27.8142, 1.6091) -> (27.6099, 2.4263)
  line L5874 (28.4681, 2.4263) -> (28.2024, 2.4263)
  line L5875 (28.2024, 2.4263) -> (28.0594, 2.2833)
  line L5876 (28.0594, 2.2833) -> (28.0594, 1.7521)
  line L5877 (28.2024, 1.6091) -> (28.0594, 1.7521)
  line L5878 (28.4681, 1.6091) -> (28.2024, 1.6091)
  line L5879 (29.122, 2.4263) -> (28.8564, 2.4263)
  line L5880 (28.8564, 2.4263) -> (28.7134, 2.2833)
  line L5881 (28.7134, 2.2833) -> (28.7134, 1.7521)
  line L5882 (28.8564, 1.6091) -> (28.7134, 1.7521)
  line L5883 (29.122, 1.6091) -> (28.8564, 1.6091)
  line L5884 (35.4255, 1.2771) -> (35.4255, 0.8684)
  line L5885 (35.3234, 0.7663) -> (35.4255, 0.8684)
  line L5886 (35.3234, 0.7663) -> (35.0781, 0.7663)
  line L5887 (35.0781, 0.7663) -> (34.976, 0.8684)
  line L5888 (34.976, 1.1749) -> (34.976, 0.8684)
  line L5889 (35.4255, 1.1749) -> (34.6082, 1.1749)
  line L5890 (34.6082, 1.2771) -> (34.6082, 0.8684)
  line L5891 (34.7103, 0.7663) -> (34.6082, 0.8684)
  line L5892 (34.8739, 0.7663) -> (34.7103, 0.7663)
  line L5893 (34.8739, 0.7663) -> (34.976, 0.8684)
  line L5894 (35.4255, 0.521) -> (34.6082, 0.521)
  line L5895 (35.4255, 0.521) -> (35.4255, 0.1124)
  line L5896 (35.4255, -0.1327) -> (34.6082, -0.1327)
  line L5897 (34.6082, -0.5417) -> (35.0169, -0.1327)
  line L5898 (35.4255, -0.5417) -> (35.0169, -0.1327)
  line L5899 (2.9373, 33.3312) -> (2.9373, 31.0325)
  line L5900 (1.7878, 32.1817) -> (4.0865, 32.1817)
  circle A0 centre (2.9372, 32.1817) radius 1.1494
  line L5901 (2.9373, 2.9373) -> (2.9373, 0.6385)
  line L5902 (1.7878, 1.7878) -> (4.0865, 1.7878)
  circle A1 centre (2.9372, 1.7878) radius 1.1495
  line L5903 (51.2099, 2.9373) -> (51.2099, 0.6385)
  line L5904 (50.0605, 1.7878) -> (52.3592, 1.7878)
  circle A2 centre (51.2099, 1.7878) radius 1.1495
  line L5905 (51.2099, 33.3312) -> (51.2099, 31.0325)
  line L5906 (50.0605, 32.1817) -> (52.3592, 32.1817)
  circle A3 centre (51.2099, 32.1817) radius 1.1494
  line L5907 (41.3772, 17.1863) -> (56.6903, 17.1863)
  line L5908 (41.3772, 6.2831) -> (56.6903, 6.2831)
  point P0 (0, 0)
  dimension "d1" = 45.974
  dimension "d20" = 3.2949
  dimension "d21" = 10.9032
  constraints: 1402 end point, 8 perpendicular, 4 midpoint, 2 parallel, 2 vertical alignment, 5218 other
  measures "d1" distance of L2168.start L2168.end
  measures "d20" distance from line of L1113.end L5908
  measures "d21" distance between parallel lines of L5908 L5907